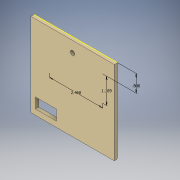
# Autodesk Inventor part: nEW bASE
Saved by Autodesk Inventor 2016 (Build 200138000, 138)
## iProperties
Created: 2017-09-12
Part Number: nEW bASE
Material: Generic
Document SubType Name: Modeling
Designer: student
Density: 1 g/cm^3
Appearance: Default
Author: student
Autodesk Inventor part; units mm, degrees
ref_plane "YZ Plane" through (0, 0, 0) normal (1, 0, 0) x (0, 1, 0)
ref_plane "XZ Plane" through (0, 0, 0) normal (0, 1, 0) x (-1, 0, 0)
ref_plane "XY Plane" through (0, 0, 0) normal (0, 0, 1) x (1, 0, 0)
sketch "Sketch1" plane through (0, 0, 0) normal (0, 0, 1) x (1, 0, 0)
  line L0 (0, 0) -> (-99.06, 0)
  line L1 (-99.06, 0) -> (-99.06, 99.06)
  line L2 (-99.06, 99.06) -> (0, 99.06)
  line L3 (0, 99.06) -> (0, 0)
  circle A0 centre (-49.53, 86.3053) radius 2.54
  line L4 (-93.599, 6.604) -> (-68.58, 6.604)
  line L5 (-68.58, 6.604) -> (-68.58, 18.8468)
  line L6 (-68.58, 18.8468) -> (-93.599, 18.8468)
  line L7 (-93.599, 18.8468) -> (-93.599, 6.604)
  point P0 (-49.53, 99.06)
  dimension "d0" = 99.06
  dimension "d1" = 99.06
  dimension "d2" = 5.08
  dimension "d16" = 25.019
  dimension "d17" = 12.2428
  dimension "d18" = 5.461
  dimension "d19" = 6.604
  dimension "d20" = 12.7547
  constraints: 16 end point, 4 parallel, 2 horizontal, 2 perpendicular, 1 centre point, 1 midpoint, 1 vertical alignment
  measures "d0" distance of L1.end L2.end
  measures "d1" distance of L0.end L1.end
  measures "d2" diameter of A0
  measures "d16" distance of L5.end L6.end
  measures "d17" distance of L4.end L5.end
  measures "d18" distance between parallel lines of L1 L7
  measures "d19" distance between parallel lines of L0 L4
  measures "d20" distance from line of L2 A0.centre
extrude "Extrusion1" add sketch "Sketch1" along normal blind 3.81
sketch "Sketch2" plane through (0, 0, 0) normal (0, 0, -1) x (-1, 0, 0)
  line L0 (0, 0) -> (99.06, 0) projected
  line L1 (99.06, 0) -> (99.06, 99.06) projected
  line L2 (50.1142, 24.5801) -> (64.0842, 24.5801)
  line L3 (64.0842, 24.5801) -> (64.0842, 46.5511)
  line L4 (64.0842, 46.5511) -> (50.1142, 46.5511)
  line L5 (50.1142, 46.5511) -> (50.1142, 24.5801)
  line L6 (48.9458, 24.5785) -> (34.9758, 24.5785)
  line L7 (34.9758, 24.5785) -> (34.9758, 46.5495)
  line L8 (34.9758, 46.5495) -> (48.9458, 46.5495)
  line L9 (48.9458, 46.5495) -> (48.9458, 24.5785)
  line L10 (50.1142, 46.5511) -> (48.7841, 46.5511) construction
  line L11 (50.1142, 35.5656) -> (48.9458, 35.564) construction
  point P0 (49.53, 35.5648)
  point P1 (49.53, 0)
  dimension "d5" = 13.97
  dimension "d6" = 21.971
  dimension "d8" = 13.97
  dimension "d9" = 21.971
  dimension "d15" = 1.1684
  constraints: 20 end point, 4 midpoint, 4 parallel, 3 horizontal, 2 perpendicular, 1 vertical alignment
  measures "d5" distance of L4.end L3.end
  measures "d6" distance of L3.end L2.end
  measures "d8" distance of L7.end L8.end
  measures "d9" distance of L6.end L7.end
  measures "d15" distance between parallel lines of L5 L9
extrude "Extrusion2" add sketch "Sketch2" along normal blind 13.97
sketch "Sketch3" plane through (0, 0, 0) normal (0, 0, -1) x (-1, 0, 0)
  line L0 (80.5561, 78.74) -> (17.8689, 78.74)
  line L1 (17.8689, 78.74) -> (17.8689, 48.5394)
  line L2 (17.8689, 48.5394) -> (80.5561, 48.5394)
  line L3 (80.5561, 48.5394) -> (80.5561, 78.74)
  line L4 (80.5561, 78.74) -> (17.8689, 48.5394) construction
  line L5 (17.8689, 78.74) -> (80.5561, 48.5394) construction
  line L6 (99.06, 99.06) -> (0, 99.06) projected
  point P0 (0, 0)
  point P1 (49.2125, 63.6397)
  dimension "d12" = 62.6872
  dimension "d13" = 30.2006
  dimension "d14" = 20.32
  constraints: 12 end point, 2 midpoint, 2 parallel, 1 horizontal, 1 perpendicular
  measures "d12" distance of L2.end L1.end
  measures "d13" distance of L1.end L0.end
  measures "d14" distance between parallel lines of L6 L0
body "Solid1"
